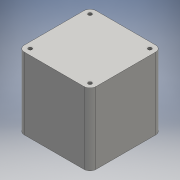
# Autodesk Inventor part: 60x60CameraMount
Saved by Autodesk Inventor 2016 (Build 200138000, 138)
## iProperties
Created: 2016-05-22
Part Number: 60x60CameraMount
Material: Generic
Document SubType Name: Modeling
Designer: Kurtis
Density: 1 g/cm^3
Appearance: Default
Author: Kurtis
Autodesk Inventor part; units mm, degrees
ref_plane "YZ Plane" through (0, 0, 0) normal (1, 0, 0) x (0, 1, 0)
ref_plane "XZ Plane" through (0, 0, 0) normal (0, 1, 0) x (-1, 0, 0)
ref_plane "XY Plane" through (0, 0, 0) normal (0, 0, 1) x (1, 0, 0)
sketch "Sketch1" plane through (0, 0, 0) normal (0, 0, 1) x (1, 0, 0)
  line L0 (-30, -30) -> (30, -30)
  line L1 (30, -30) -> (30, 30)
  line L2 (30, 30) -> (-30, 30)
  line L3 (-30, 30) -> (-30, -30)
  line L4 (-30, -30) -> (30, 30) construction
  line L5 (30, -30) -> (-30, 30) construction
  line L6 (30, 30) -> (25, 30) construction
  line L7 (25, 30) -> (25, 25) construction
  line L8 (-30, 30) -> (-25, 30) construction
  line L9 (-25, 30) -> (-25, 25) construction
  line L10 (-30, -30) -> (-30, -25) construction
  line L11 (-30, -25) -> (-25, -25) construction
  line L12 (30, -30) -> (30, -25) construction
  line L13 (30, -25) -> (25, -25) construction
  circle A0 centre (-25, 25) radius 1.5
  circle A1 centre (25, 25) radius 1.5
  circle A2 centre (25, -25) radius 1.5
  circle A3 centre (-25, -25) radius 1.5
  point P0 (0, 0)
  dimension "d0" = 60
  dimension "d1" = 60
  dimension "d2" = 5
  dimension "d3" = 5
  dimension "d4" = 5
  dimension "d5" = 5
  dimension "d6" = 5
  dimension "d7" = 5
  dimension "d8" = 5
  dimension "d9" = 5
  dimension "d10" = 3
  dimension "d11" = 3
  dimension "d12" = 3
  dimension "d13" = 3
  constraints: 28 end point, 8 point on line, 4 centre point, 4 coincident, 2 midpoint, 2 parallel, 1 horizontal, 1 perpendicular
  measures "d0" distance of L2.end L1.end
  measures "d1" distance of L1.end L0.end
  measures "d2" distance of L1.end L6.end
  measures "d3" distance of L6.end L7.end
  measures "d4" distance of L2.end L8.end
  measures "d5" distance of L8.end L9.end
  measures "d6" distance of L0.start L10.end
  measures "d7" distance of L10.end L11.end
  measures "d8" distance of L0.end L12.end
  measures "d9" distance of L12.end L13.end
  measures "d10" diameter of A0
  measures "d11" diameter of A1
  measures "d12" diameter of A2
  measures "d13" diameter of A3
extrude "Block" add sketch "Sketch1" along normal blind 60
fillet "Fillets FTW" radius 5 4 edges at (-30, 30, 30) (-30, -30, 30) (30, -30, 30) (30, 30, 30)
body "Solid1"
